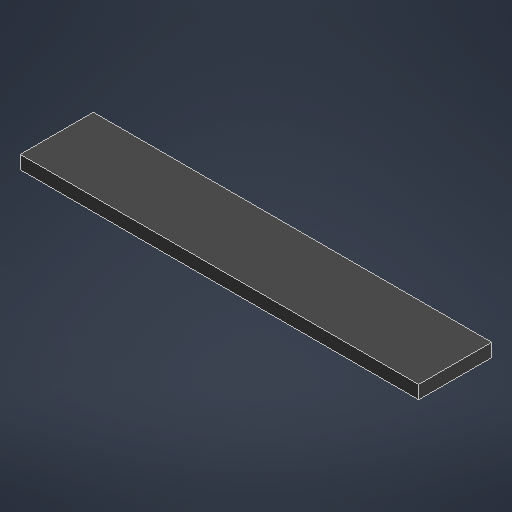
# Autodesk Inventor part: P_Spacer_Dummy_ESP32C3
Saved by Autodesk Inventor 2026 (Build 300175000, 175)
## iProperties
Created: 2025-09-06
Part Number: P_Spacer_Dummy_ESP32C3
Material: Generisch
Document SubType Name: Modeling
Designer: FAL
Density: 1 g/cm^3
Appearance: Vorgabe
Author: FAL
Autodesk Inventor part; units mm, degrees
ref_plane "YZ Plane" through (0, 0, 0) normal (1, 0, 0) x (0, 1, 0)
ref_plane "XZ Plane" through (0, 0, 0) normal (0, 1, 0) x (-1, 0, 0)
ref_plane "XY Plane" through (0, 0, 0) normal (0, 0, 1) x (1, 0, 0)
sketch "Skizze1" plane through (0, 0, 0) normal (0, 1, 0) x (-1, 0, 0)
  line L0 (-30, -1) -> (30, -1)
  line L1 (30, -1) -> (30, 1)
  line L2 (30, 1) -> (-30, 1)
  line L3 (-30, 1) -> (-30, -1)
  line L4 (-30, -1) -> (30, 1) construction
  line L5 (30, -1) -> (-30, 1) construction
  point P0 (0, 0)
  dimension "d0" = 2
  dimension "d3" = 60
  constraints: 12 end point, 2 midpoint, 2 parallel, 1 horizontal, 1 perpendicular
  measures "d0" distance between parallel lines of L0 L2
  measures "d3" distance of L1.end L2.end
extrude "Extrusion1" add sketch "Skizze1" along normal blind 11
